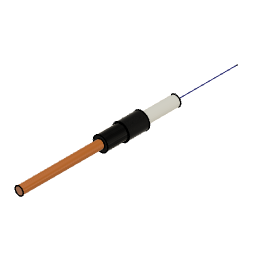
Linear motivated UV DIB CAD design (Autodesk Fusion 360 archive; units mm, degrees)
design "Fibre Optic"
Autodesk Fusion 360 part; units mm, degrees
sketch "Real Dimensions" plane through (0, 0, 0) normal (0, 0, 1) x (1, 0, 0)
  line L0 (0, 0) -> (2.5, 0)
  line L1 (2.5, 0) -> (2.5, -8.4)
  line L2 (2.5, -8.4) -> (0, -8.4)
  line L3 (0, -8.4) -> (0, 0)
  line L4 (2.5, -8.4) -> (3.25, -8.4)
  line L5 (0, -8.4) -> (-0.75, -8.4)
  line L6 (-0.75, -8.4) -> (-0.75, -13.4)
  line L7 (3.25, -8.4) -> (3.25, -13.4)
  line L8 (-0.75, -13.4) -> (3.25, -13.4)
  line L9 (1.25, -13.4) -> (3, -13.4)
  line L10 (3, -13.4) -> (3, -18.4)
  line L11 (3, -18.4) -> (-0.5, -18.4)
  line L12 (-0.5, -18.4) -> (-0.5, -13.4)
  line L13 (1.25, -18.4) -> (0.25, -18.4)
  line L14 (0.25, -18.4) -> (0.25, -38.4)
  line L15 (0.25, -38.4) -> (2.25, -38.4)
  line L16 (2.25, -38.4) -> (2.25, -18.4)
  line L17 (1.25, 0) -> (1.25, -38.4)
  dimension "d1" = 2.5
  dimension "d2" = 8.4
  dimension "d3" = 0.75
  dimension "d4" = 0.75
  dimension "d5" = 5
  dimension "d6" = 5
  dimension "d7" = 1.75
  dimension "d8" = 5
  dimension "d9" = 3.5
  dimension "d10" = 1
  dimension "d11" = 20
  dimension "d12" = 2
  constraint horizontal L0
  constraint vertical L1
  constraint horizontal L2
  constraint vertical L3
  constraint coincident L0.start L3.end
  constraint perpendicular L1 L4
  constraint perpendicular L3 L5
  constraint perpendicular L5 L6
  constraint perpendicular L4 L7
  constraint midpoint L8 L9.start
  constraint perpendicular L6 L9
  constraint perpendicular L8 L10
  constraint perpendicular L10 L11
  constraint coincident L8 L12.end
  constraint perpendicular L8 L12
  constraint midpoint L11 L13.start
  constraint perpendicular L12 L13
  constraint perpendicular L13 L14
  constraint perpendicular L14 L15
  constraint coincident L11 L16.end
  constraint perpendicular L11 L16
  constraint midpoint L0 L17.start
  constraint midpoint L15 L17.end
  measures "d1" distance of L0.start L0.end
  measures "d2" distance of L0.start L2.end
  measures "d3" distance of L1.end L4.end
  measures "d4" distance of L2.end L5.end
  measures "d5" distance of L5.end L6.end
  measures "d6" distance of L4.end L7.end
  measures "d7" distance of L9.start L9.end
  measures "d8" distance of L9.end L10.end
  measures "d9" distance of L10.end L11.end
  measures "d10" distance of L13.start L13.end
  measures "d11" distance of L13.end L14.end
  measures "d12" distance of L14.end L15.end
sketch "Sketch2" plane through (0, 0, 0) normal (0, 0, 1) x (1, 0, 0)
  line L0 (1.25, -8.4) -> (0, -8.4)
  line L1 (0, -8.4) -> (0, 0)
  line L2 (1.25, 0) -> (1.25, -8.4)
  line L3 (0, 0) -> (1.25, 0)
  line L4 (1.25, -8.4) -> (1.625, -8.4)
  line L5 (0, -8.4) -> (-0.375, -8.4)
  line L6 (-0.375, -8.4) -> (-0.375, -13.4)
  line L7 (-0.375, -13.4) -> (1.625, -13.4)
  line L8 (1.625, -13.4) -> (1.625, -8.4)
  line L9 (0.625, -13.4) -> (-0.25, -13.4)
  line L10 (-0.25, -13.4) -> (-0.25, -18.4)
  line L11 (-0.25, -18.4) -> (1.5, -18.4)
  line L12 (1.5, -18.4) -> (1.5, -13.4)
  line L13 (0.625, -18.4) -> (0.125, -18.4)
  line L14 (0.125, -18.4) -> (0.125, -28.4)
  line L15 (0.125, -28.4) -> (1.125, -28.4)
  line L16 (1.125, -28.4) -> (1.125, -18.4)
  dimension "d13" = 1.25
  dimension "d14" = 8.4
  dimension "d25" = 0.375
  dimension "d26" = 0.375
  dimension "d27" = 5
  dimension "d28" = 2
  dimension "d29" = 0.875
  dimension "d30" = 5
  dimension "d31" = 1.75
  dimension "d32" = 0.5
  dimension "d33" = 10
  dimension "d34" = 1
  constraint horizontal L3
  constraint vertical L2
  constraint horizontal L0
  constraint vertical L1
  constraint coincident L1.end L3.start
  constraint perpendicular L2 L4
  constraint perpendicular L1 L5
  constraint perpendicular L5 L6
  constraint perpendicular L6 L7
  constraint midpoint L7 L9.start
  constraint parallel L7 L9
  constraint perpendicular L9 L10
  constraint perpendicular L10 L11
  constraint coincident L7 L12.end
  constraint perpendicular L7 L12
  constraint midpoint L11 L13.start
  constraint perpendicular L12 L13
  constraint perpendicular L13 L14
  constraint perpendicular L14 L15
  constraint coincident L11 L16.end
  constraint perpendicular L11 L16
  measures "d13" distance of L1.end L2.start
  measures "d14" distance of L1.end L0.end
  measures "d25" distance of L0.start L4.end
  measures "d26" distance of L0.end L5.end
  measures "d27" distance of L5.end L6.end
  measures "d28" distance of L6.end L7.end
  measures "d29" distance of L9.start L9.end
  measures "d30" distance of L9.end L10.end
  measures "d31" distance of L10.end L11.end
  measures "d32" distance of L13.start L13.end
  measures "d33" distance of L13.end L14.end
  measures "d34" distance of L14.end L15.end
revolve "Revolve3" add sketch "Real Dimensions" angle 360 about axis through (1.25, 0, 0) along (0, -1, 0) contours L0 L1 L2 L17 makes body 1
revolve "Revolve4" add sketch "Real Dimensions" angle 360 about axis through (1.25, 0, 0) along (0, -1, 0) contours L2 L4 L7 L8 L9 L17 bodies 1
revolve "Revolve5" add sketch "Real Dimensions" angle 360 about axis through (1.25, 0, 0) along (0, -1, 0) contours L8 L9 L10 L11 L17 bodies 1
revolve "Revolve6" add sketch "Real Dimensions" angle 360 about axis through (1.25, 0, 0) along (0, -1, 0) contours L11 L15 L16 L17 bodies 1
hole "Hole1" at (1.25, 0, 0) direction (0, -1, 0) diameter 0.1 depth 1 tip angle 118 bodies 1
move_body "Move1" bodies 1 to x (1, 0, 0) y (0, 1, 0) z (0, 0, 1) at (0, 0, -0.5)
move_body "Move2" bodies 1 to x (1, 0, 0) y (0, 1, 0) z (0, 0, 1) at (-66, 0, -8)
move_body "Move3" bodies 1 to x (1, 0, 0) y (0, 1, 0) z (0, 0, 1) at (66, 0, 8)
cylinder "CylinderPrimitive1" add diameter 0.2 height 15 placed x (-1, 0, 0) y (0, 0, 1) z (0, 1, 0) at (1.25, 0, -0.5) separate body makes body 2
